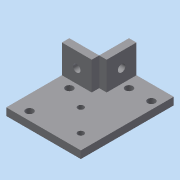
# Autodesk Inventor part: Corner Mount
Saved by Autodesk Inventor 2015 (Build 190159000, 159)
## iProperties
Created: 2016-09-07
Part Number: Corner Mount
Material: Generic
Document SubType Name: Modeling
Designer: Dustin
Density: 1 g/cm^3
Appearance: Default
Author: Dustin
Autodesk Inventor part; units mm, degrees
ref_plane "YZ Plane" through (0, 0, 0) normal (1, 0, 0) x (0, 1, 0)
ref_plane "XZ Plane" through (0, 0, 0) normal (0, 1, 0) x (-1, 0, 0)
ref_plane "XY Plane" through (0, 0, 0) normal (0, 0, 1) x (1, 0, 0)
sketch "Sketch1" plane through (0, 0, 0) normal (0, 0, 1) x (1, 0, 0)
  line L0 (0, 0) -> (30, 0)
  line L1 (30, 0) -> (30, 42.3)
  line L2 (30, 42.3) -> (0, 42.3)
  line L3 (0, 42.3) -> (0, 0)
  line L4 (0, 0.3) -> (0, 42.3)
  line L5 (0, 42.3) -> (42.3, 42.3)
  line L6 (0, 42.3) -> (30, 42.3)
  line L7 (30, 42.3) -> (30, 62.3)
  line L8 (30, 62.3) -> (0, 62.3)
  line L9 (0, 62.3) -> (0, 42.3)
  line L10 (0, 42.3) -> (-20, 42.3)
  line L11 (-20, 42.3) -> (-20, 0)
  line L12 (-20, 0) -> (0, 0)
  line L13 (0, 0) -> (0, 42.3)
  point P0 (10, 52.3)
  point P1 (25, 52.3)
  point P2 (-10, 32.3)
  point P3 (-10, 5.65)
  dimension "d0" = 30
  dimension "d16" = 42.3
  dimension "d21" = 20
  dimension "d22" = 20
  dimension "d49" = 30
  dimension "d50" = 5
  dimension "d69" = 10
  dimension "d70" = 10
  dimension "d71" = 10
  constraints: 28 end point, 6 parallel, 4 horizontal, 3 perpendicular
  measures "d0" distance of L1.end L2.end
  measures "d16" distance of L2.end L0.start
  measures "d21" distance of L6.end L7.end
  measures "d22" distance of L2.end L10.end
  measures "d49" distance of L7.end L8.end
  measures "d50" distance from line of L7 point (25, 52.3)
  measures "d69" distance from line of L10 point (-10, 32.3)
  measures "d70" distance from line of L4 point (-10, 32.3)
  measures "d71" distance from line of L9 point (10, 52.3)
extrude "Extrusion1" [suppressed]
hole "Hole2" [suppressed]
extrude "Extrusion2" add sketch "Sketch1" along normal blind 5
hole "Hole3" at (25, 52.3, 0) at (10, 52.3, 0) at (-10, 32.3, 0) at (-10, 5.65, 0) direction (0, 0, 1) diameter 5 depth 8 tip angle 118
sketch "Sketch2" plane through (0, 0, 0) normal (0, 0, -1) x (-1, 0, 0)
  line L0 (20, 0) -> (-30, 0) projected
  line L1 (-30, 0) -> (-30, 62.3) projected
  point P0 (0, 0)
  point P1 (-20, 10)
  dimension "d51" = 10
  dimension "d52" = 10
  measures "d51" distance from line of L0 point (-20, 10)
  measures "d52" distance from line of point (-20, 10) L1
hole "Hole4" at (20, 10, 0) direction (0, 0, 1) diameter 4 depth 8 tip angle 118
sketch "Sketch3" plane through (0, 0, 0) normal (0, 0, -1) x (-1, 0, 0)
  line L0 (-30, 0) -> (-30, 62.3) projected
  line L1 (20, 0) -> (-30, 0) projected
  point P0 (0, 0)
  point P1 (-5, 25)
  dimension "d60" = 25
  dimension "d61" = 25
  measures "d60" distance from line of L0 point (-5, 25)
  measures "d61" distance from line of L1 point (-5, 25)
hole "Hole5" at (5, 25, 0) direction (0, 0, 1) diameter 4 depth 8 tip angle 118
sketch "Sketch4" plane through (0, 0, 5) normal (0, 0, 1) x (1, 0, 0)
  line L0 (-20, 42.3) -> (0, 42.3)
  line L1 (0, 42.3) -> (0, 37.3)
  line L2 (0, 37.3) -> (-20, 37.3)
  line L3 (-20, 37.3) -> (-20, 42.3)
  line L4 (30, 62.3) -> (0, 62.3) projected
  line L5 (0, 42.3) -> (5, 42.3)
  line L6 (5, 42.3) -> (5, 62.3)
  line L7 (5, 62.3) -> (0, 62.3)
  line L8 (0, 62.3) -> (0, 42.3)
  point P0 (0, 0)
  dimension "d72" = 5
  dimension "d73" = 5
  constraints: 16 end point, 4 parallel, 2 horizontal, 2 perpendicular, 1 point on line
  measures "d72" distance between parallel lines of L8 L6
  measures "d73" distance of L0.end L1.end
extrude "Extrusion3" add sketch "Sketch4" along normal blind 19
sketch "Sketch5" plane through (-20, 37.3, 5) normal (0, -1, 0) x (1, 0, 0)
  line L0 (20, 19) -> (0, 19) projected
  line L1 (0, -5) -> (0, 19) projected
  point P0 (20, -5)
  point P1 (10, 9)
  dimension "d76" = 10
  dimension "d77" = 10
  measures "d76" distance from line of L0 point (10, 9)
  measures "d77" distance from line of L1 point (10, 9)
hole "Hole6" at (-10, 37.3, 14) direction (0, 1, 0) diameter 5 depth 8 tip angle 118
sketch "Sketch6" plane through (5, 42.3, 5) normal (1, 0, 0) x (0, 0, -1)
  line L0 (-19, 20) -> (-19, 0) projected
  line L1 (5, 20) -> (-19, 20) projected
  point P0 (5, -42.3)
  point P1 (-9, 10)
  dimension "d85" = 10
  dimension "d86" = 10
  measures "d85" distance from line of L0 point (-9, 10)
  measures "d86" distance from line of L1 point (-9, 10)
hole "Hole7" at (5, 52.3, 14) direction (-1, 0, 0) diameter 5 depth 8 tip angle 118
body "Solid1"
